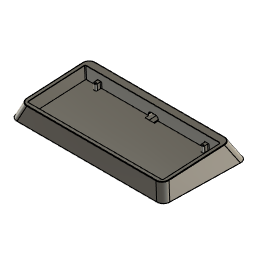
Bruce the Menhir Bottom Mount (Autodesk Fusion 360 design; units mm, degrees)
Autodesk Fusion 360 part; units mm, degrees
sketch "Top Plane Sketch" plane through (0, 0, 0) normal (0, 0, 1) x (1, 0, 0)
  line L0 (-95.25, -40.4812) -> (95.25, -40.4812) construction
  line L1 (95.25, -40.4812) -> (95.25, 40.4812) construction
  line L2 (95.25, 40.4812) -> (-95.25, 40.4812) construction
  line L3 (-95.25, 40.4812) -> (-95.25, -40.4812) construction
  line L4 (-95.75, -40.9812) -> (95.75, -40.9812)
  line L5 (95.75, -40.9812) -> (95.75, 40.9812)
  line L6 (95.75, 40.9813) -> (-95.75, 40.9813)
  line L7 (-95.75, 40.9813) -> (-95.75, -40.9812)
  line L8 (-100.75, -45.9812) -> (100.75, -45.9812)
  line L9 (100.75, -45.9812) -> (100.75, 50.9812)
  line L10 (100.75, 50.9813) -> (-100.75, 50.9813)
  line L11 (-100.75, 50.9813) -> (-100.75, -45.9812)
  line L12 (-95.25, 40.4812) -> (95.25, -40.4812) construction
  line L13 (95.25, 40.4812) -> (-95.25, -40.4812) construction
  circle A0 centre (0, 0) radius 1.8249 construction
  dimension "d1" = 190.5
  dimension "d2" = 80.9625
  dimension "d3" = 0.5
  dimension "d9" = 10
  dimension "d10" = 5
  dimension "d11" = 5
  dimension "d12" = 5
  constraint horizontal L0
  constraint vertical L1
  constraint horizontal L2
  constraint vertical L3
  constraint midpoint L12 A0.centre
  measures "d1" distance of L0.start L0.end
  measures "d2" distance of L0.start L2.end
  measures "d9" distance of L6 L10
  measures "d10" distance of L7 L11
  measures "d11" distance of L5 L9
  measures "d12" distance of L4 L8
ref_plane "WorkPlane1" through (0, 0, -50) normal (0, 0, 1) x (1, 0, 0)
sketch "Base Plane Sketch" plane through (0, 0, -50) normal (0, 0, 1) x (1, 0, 0)
  line L0 (95.25, -40.4813) -> (-95.25, -40.4813) construction
  line L1 (-95.25, -40.4813) -> (-95.25, 40.4812) construction
  line L2 (-95.25, 40.4812) -> (95.25, 40.4812) construction
  line L3 (95.25, 40.4812) -> (95.25, -40.4813) construction
  line L4 (95.25, -40.4813) -> (-95.25, 40.4813) construction
  line L5 (-95.25, -40.4813) -> (95.25, 40.4812) construction
  circle A0 centre (0, 0) radius 6.9017 construction
  line L6 (95.75, -40.9813) -> (-95.75, -40.9813) construction
  line L7 (-95.75, -40.9813) -> (-95.75, 40.9812) construction
  line L8 (-95.75, 40.9812) -> (95.75, 40.9812) construction
  line L9 (95.75, 40.9812) -> (95.75, -40.9812) construction
  line L10 (-100.75, 50.9812) -> (100.75, 50.9812) construction
  line L11 (100.75, 50.9812) -> (100.75, -45.9812) construction
  line L12 (100.75, -45.9813) -> (-100.75, -45.9813) construction
  line L13 (-100.75, -45.9813) -> (-100.75, 50.9812) construction
  line L14 (-120.75, 74.9813) -> (120.75, 74.9813)
  line L15 (120.75, 74.9813) -> (120.75, -65.9813)
  line L16 (120.75, -65.9813) -> (-120.75, -65.9812)
  line L17 (-120.75, -65.9812) -> (-120.75, 74.9812)
  dimension "d14" = 190.5
  dimension "d15" = 80.9625
  dimension "d16" = -0.5
  dimension "d17" = 10
  dimension "d18" = 5
  dimension "d19" = 5
  dimension "d20" = 5
  dimension "d21" = 20
  dimension "d22" = 20
  dimension "d23" = 20
  dimension "d24" = 24
  constraint horizontal L0
  constraint perpendicular L0 L1
  constraint parallel L0 L2
  constraint parallel L1 L3
  constraint coincident L4 A0.centre
  constraint coincident L5 A0.centre
  constraint coincident A0.centre origin
  constraint horizontal L10
  constraint vertical L11
  constraint horizontal L12
  constraint vertical L13
  constraint horizontal L14
  constraint vertical L15
  constraint horizontal L16
  constraint vertical L17
  measures "d14" distance of L1.end L2.end
  measures "d15" distance of L0.end L1.end
  measures "d17" distance of L8 L10
  measures "d18" distance of L7 L13
  measures "d19" distance of L9 L11
  measures "d20" distance of L6 L12
  measures "d21" distance of L12 L16
  measures "d22" distance of L11 L15
  measures "d23" distance of L13 L17
  measures "d24" distance of L10 L14
loft "Loft1" add profiles "Top Plane Sketch", "Base Plane Sketch" section 1 section 2
sketch "Angle Cut Line" plane through (0, -39.639, 15.8556) normal (0, -0.928477, 0.371391) x (1, 0, 0)
  line L0 (100.75, -17.077) -> (-100.75, -17.077)
  line L1 (-100.75, -17.077) -> (-120.75, -70.9287)
  line L2 (-120.75, -70.9287) -> (120.75, -70.9287)
  line L3 (120.75, -70.9287) -> (100.75, -17.077)
  line L4 (-108.5492, -38.077) -> (108.5492, -38.077)
  dimension "d37" = 21
  constraint coincident L1 L4.start
  constraint coincident L3 L4.end
  constraint parallel L2 L4
  measures "d37" distance of L0 L4
ref_plane "WorkPlane2" through (0, -53.7805, -19.498) normal (0, 0.052336, 0.99863) x (1, 0, 0)
extrude "Extrude1" cut 1 faces at (-40.25, 27.9937, -50) along direction (0, 0, -1) up to surface end surface through (0, -53.7805, -19.498) normal (0, 0.052336, 0.99863) offset 0
fillet "Fillet1" radius 10 4 edges at (-105.8766, 57.1332, -12.8166) (-104.6496, -49.8809, -9.749) (104.6496, -49.8809, -9.749) (105.8766, 57.1332, -12.8166)
extrude "Extrude2" cut sketch "Top Plane Sketch" against normal blind 18.06 contours L4 L5 L6 L7
fillet "Fillet2" radius 1 4 edges at (-95.75, 40.9813, -9.03) (95.75, 40.9813, -9.03) (95.75, -40.9812, -9.03) (-95.75, -40.9812, -9.03)
chamfer "Chamfer1" distance 0.5 angle 45 8 edges at (0, -45.9812, 0) (98.1037, -43.335, 0) (100.75, 2.4876, 0) (98.1846, 48.3392, 0) (0, 50.9813, 0) (-98.1846, 48.3392, 0) (-100.75, 2.4876, 0) (-98.1037, -43.335, 0)
chamfer "Chamfer3" distance 0.25 angle 45 8 edges at (0, 40.9813, 0) (95.4571, 40.6884, 0) (95.75, 0, 0) (95.4571, -40.6884, 0) (0, -40.9812, 0) (-95.4571, -40.6884, 0) (-95.75, 0, 0) (-95.4571, 40.6884, 0)
chamfer "Chamfer4" distance 0.5 angle 45 8 edges at (-109.7715, 4.5245, -22.5536) (-105.9572, -51.1885, -19.6338) (0, -53.7805, -19.498) (105.9572, -51.1885, -19.6338) (109.7715, 4.5245, -22.5536) (108.3811, 60.5749, -25.4911) (0, 63.2852, -25.6332) (-108.3811, 60.5749, -25.4911)
sketch "Screw Post Sketch" plane through (0, 0, -18.06) normal (0, 0, 1) x (1, 0, 0)
  arc A0 (-95.75, -39.9812) -> (-94.75, -40.9812) centre (-94.75, -39.9812) ccw
  line L0 (79.45, -40.9812) -> (94.75, -40.9812)
  arc A1 (94.75, -40.9813) -> (95.75, -39.9813) centre (94.75, -39.9813) ccw
  line L1 (95.75, -39.9813) -> (95.75, 39.9813)
  arc A2 (95.75, 39.9812) -> (94.75, 40.9813) centre (94.75, 39.9813) ccw
  line L2 (-79.45, 40.9813) -> (-94.75, 40.9813)
  arc A3 (-94.75, 40.9813) -> (-95.75, 39.9813) centre (-94.75, 39.9813) ccw
  line L3 (-95.75, 39.9813) -> (-95.75, -39.9812)
  arc A4 (-95.75, -39.9812) -> (-94.75, -40.9812) centre (-94.75, -39.9812) ccw
  line L4 (-72.95, -40.9812) -> (72.95, -40.9812)
  arc A5 (94.75, -40.9813) -> (95.75, -39.9813) centre (94.75, -39.9813) ccw
  line L5 (95.75, -39.9813) -> (95.75, 39.9813)
  arc A6 (95.75, 39.9812) -> (94.75, 40.9813) centre (94.75, 39.9813) ccw
  line L6 (72.95, 40.9813) -> (-72.95, 40.9812)
  arc A7 (-94.75, 40.9813) -> (-95.75, 39.9813) centre (-94.75, 39.9813) ccw
  line L7 (-95.75, 39.9813) -> (-95.75, -39.9812)
  arc A8 (-95.75, -39.9812) -> (-94.75, -40.9812) centre (-94.75, -39.9812) ccw
  line L8 (-94.75, -40.9812) -> (94.75, -40.9812)
  arc A9 (94.75, -40.9813) -> (95.75, -39.9813) centre (94.75, -39.9813) ccw
  line L9 (95.75, -39.9813) -> (95.75, 39.9813)
  arc A10 (95.75, 39.9812) -> (94.75, 40.9813) centre (94.75, 39.9813) ccw
  line L10 (94.75, 40.9813) -> (-94.75, 40.9813)
  arc A11 (-94.75, 40.9813) -> (-95.75, 39.9813) centre (-94.75, 39.9813) ccw
  line L11 (-95.75, 39.9813) -> (-95.75, -39.9812)
  line L12 (-95.25, 39.9813) -> (-95.25, -39.9812) construction
  arc A12 (-95.25, -39.9812) -> (-94.75, -40.4812) centre (-94.75, -39.9812) ccw construction
  line L13 (-94.75, -40.4812) -> (94.75, -40.4812) construction
  arc A13 (94.75, -40.4813) -> (95.25, -39.9813) centre (94.75, -39.9813) ccw construction
  line L14 (95.25, -39.9813) -> (95.25, 39.9813) construction
  arc A14 (95.25, 39.9812) -> (94.75, 40.4812) centre (94.75, 39.9813) ccw construction
  line L15 (94.75, 40.4812) -> (-94.75, 40.4813) construction
  arc A15 (-94.75, 40.4813) -> (-95.25, 39.9813) centre (-94.75, 39.9813) ccw construction
  circle A16 centre (-76.2, 35.7187) radius 1
  circle A17 centre (76.2, 35.7187) radius 1
  circle A18 centre (-76.2, -35.7187) radius 1
  circle A19 centre (76.2, -35.7187) radius 1
  circle A20 centre (-76.2, 35.7187) radius 2.25
  circle A21 centre (76.2, 35.7187) radius 2.25
  circle A22 centre (76.2, -35.7187) radius 2.25
  circle A23 centre (-76.2, -35.7187) radius 2.25
  line L16 (-78.45, 35.7187) -> (-78.45, 39.9813)
  line L17 (-73.95, 35.7187) -> (-73.95, 39.9813)
  line L18 (-78.45, -35.7187) -> (-78.45, -39.9812)
  line L19 (-73.95, -35.7187) -> (-73.95, -39.9812)
  line L20 (78.45, -35.7187) -> (78.45, -39.9812)
  line L21 (73.95, -35.7187) -> (73.95, -39.9812)
  line L22 (73.95, 35.7187) -> (73.95, 39.9813)
  line L23 (78.45, 35.7187) -> (78.45, 39.9813)
  arc A24 (-78.45, 39.9813) -> (-79.45, 40.9812) centre (-79.45, 39.9813) ccw
  arc A25 (-72.95, 40.9812) -> (-73.95, 39.9813) centre (-72.95, 39.9813) ccw
  arc A26 (73.95, 39.9813) -> (72.95, 40.9812) centre (72.95, 39.9813) ccw
  arc A27 (79.45, 40.9812) -> (78.45, 39.9813) centre (79.45, 39.9813) ccw
  arc A28 (78.45, -39.9812) -> (79.45, -40.9813) centre (79.45, -39.9812) ccw
  arc A29 (72.95, -40.9812) -> (73.95, -39.9812) centre (72.95, -39.9812) ccw
  arc A30 (-73.95, -39.9812) -> (-72.95, -40.9812) centre (-72.95, -39.9812) ccw
  arc A31 (-79.45, -40.9812) -> (-78.45, -39.9812) centre (-79.45, -39.9813) ccw
  dimension "d80" = 2
  dimension "d81" = 19.05
  dimension "d82" = 2
  dimension "d83" = 2
  dimension "d84" = 2
  dimension "d85" = 19.05
  dimension "d86" = 19.05
  dimension "d87" = 19.05
  dimension "d88" = 4.7625
  dimension "d89" = 4.7625
  dimension "d90" = 4.7625
  dimension "d91" = 4.7625
  dimension "d92" = 4.5
  dimension "d93" = 4.5
  dimension "d94" = 4.5
  dimension "d95" = 4.5
  dimension "d96" = 1
  dimension "d97" = 1
  dimension "d98" = 1
  dimension "d99" = 1
  dimension "d100" = 1
  constraint concentric A16 A20
  constraint concentric A17 A21
  constraint concentric A19 A22
  constraint concentric A18 A23
  constraint coincident A20 L16.start
  constraint tangent A20 L16
  constraint perpendicular L10 L16
  constraint coincident A20 L17.start
  constraint tangent A20 L17
  constraint perpendicular L6 L17
  constraint coincident A23 L18.start
  constraint tangent A23 L18
  constraint perpendicular L4 L18
  constraint coincident A23 L19.start
  constraint tangent A23 L19
  constraint perpendicular L4 L19
  constraint coincident A22 L20.start
  constraint tangent A22 L20
  constraint perpendicular L4 L20
  constraint coincident A22 L21.start
  constraint tangent A22 L21
  constraint perpendicular L0 L21
  constraint coincident A21 L22.start
  constraint tangent A21 L22
  constraint perpendicular L10 L22
  constraint coincident A21 L23.start
  constraint tangent A21 L23
  constraint perpendicular L2 L23
  constraint concentric A0 A12
  constraint concentric A1 A13
  constraint concentric A2 A14
  constraint concentric A3 A15
  constraint tangent A13 L14
  constraint tangent A12 L13
  constraint tangent L12 A15
  constraint tangent L12 A12
  constraint tangent A14 L15
  constraint tangent L13 A13
  constraint tangent L15 A15
  constraint tangent L14 A14
  constraint tangent L2 A24
  constraint tangent L16 A24
  constraint tangent L17 A25
  constraint tangent L6 A25
  constraint equal A24 A25
  constraint tangent L6 A26
  constraint tangent L22 A26
  constraint tangent L23 A27
  constraint tangent L20 A28
  constraint tangent L0 A28
  constraint tangent L21 A29
  constraint tangent L4 A29
  constraint equal A28 A29
  constraint tangent L19 A30
  constraint tangent L4 A30
  constraint equal A28 A30
  constraint tangent L18 A31
  measures "d80" diameter of A16
  measures "d81" distance of L12 A16.centre
  measures "d82" diameter of A17
  measures "d83" diameter of A18
  measures "d84" diameter of A19
  measures "d85" distance of L12 A18.centre
  measures "d86" distance of L14 A19.centre
  measures "d87" distance of L14 A17.centre
  measures "d88" distance of L15 A16.centre
  measures "d89" distance of L15 A17.centre
  measures "d90" distance of L13 A19.centre
  measures "d91" distance of L13 A18.centre
  measures "d92" diameter of A20
  measures "d93" diameter of A21
  measures "d94" diameter of A22
  measures "d95" diameter of A23
  measures "d96" radius of A24
  measures "d97" radius of A26
  measures "d98" radius of A27
  measures "d99" radius of A28
  measures "d100" radius of A31
extrude "Extrude4" add sketch "Screw Post Sketch" along normal blind 8.41 contours L8 A23 L18 L19 A30 A31 | L10 A20 L16 L17 A24 A25 | L8 A22 L20 L21 A28 A29 | A23 | L10 A21 L22 L23 A26 A27 | A20 | A22 | A21
sketch "USB C Hole" plane through (0, 40.9813, 0) normal (0, -1, 0) x (1, 0, 0)
  line L0 (94.75, -0.25) -> (-94.75, -0.25)
  line L1 (-94.75, -0.25) -> (-94.75, -18.06)
  line L2 (94.75, -18.06) -> (94.75, -0.25)
  line L3 (0, -18.06) -> (0, -16.23) construction
  line L4 (6.975, -12.15) -> (-6.975, -12.15)
  line L5 (-6.975, -12.15) -> (-6.975, -20.31)
  line L6 (-6.975, -20.31) -> (6.975, -20.31)
  line L7 (6.975, -20.31) -> (6.975, -12.15)
  line L8 (6.975, -12.15) -> (-6.975, -20.31) construction
  line L9 (-6.975, -12.15) -> (6.975, -20.31) construction
  line L10 (72.95, -9.65) -> (79.45, -9.65)
  line L11 (79.45, -18.06) -> (94.75, -18.06)
  line L12 (-79.45, -18.06) -> (-79.45, -9.65)
  line L13 (-72.95, -9.65) -> (-72.95, -18.06)
  line L14 (-72.95, -18.06) -> (72.95, -18.06)
  line L15 (72.95, -18.06) -> (72.95, -9.65)
  line L16 (79.45, -9.65) -> (79.45, -18.06)
  line L17 (-79.45, -9.65) -> (-72.95, -9.65)
  line L18 (-94.75, -18.06) -> (-79.45, -18.06)
  line L19 (-94.75, -18.06) -> (0, -18.06)
  line L20 (-6.975, -16.23) -> (6.975, -16.23) construction
  point P0 (0, -16.23)
  dimension "d60" = 1.83
  dimension "d61" = 13.95
  dimension "d62" = 8.16
  constraint horizontal L4
  constraint perpendicular L4 L5
  constraint parallel L4 L6
  constraint parallel L5 L7
  constraint coincident L8 P0
  constraint coincident L9 P0
  constraint coincident P0 L3.end
  constraint coincident L1.end L18.start
  constraint midpoint L14 L3.start
  constraint midpoint L5 L20.start
  constraint midpoint L7 L20.end
  constraint perpendicular L3 L20
  constraint coincident L3.start L19.end
  measures "d60" distance of L3.start P0
  measures "d61" distance of L5.end L6.end
  measures "d62" distance of L4.end L5.end
extrude "Extrude5" cut sketch "USB C Hole" along normal blind -25 and the other way blind -5 contours L5 L6 L7 L14 L19 | L4 L5 L7 L14 L19
fillet "Fillet3" radius 3.8 4 edges at (6.975, 48.3557, -20.31) (6.975, 48.8973, -12.15) (-6.975, 48.3557, -20.31) (-6.975, 48.8973, -12.15)
chamfer "Chamfer5" distance 0.25 angle 45 8 edges at (0, 56.8133, -12.15) (-5.862, 57.3475, -13.263) (-6.975, 58.7717, -16.23) (-5.862, 60.1958, -19.197) (0, 60.7301, -20.31) (5.862, 60.1958, -19.197) (6.975, 58.7717, -16.23) (5.862, 57.3475, -13.263)
move_body "Move2" bodies 1 to x (1, 0, 0) y (0, 0.99863, 0.052336) z (0, -0.052336, 0.99863) at (0, -1.0948, 2.7618)
equation "d1 = 19.05 mm * 10"
equation "d2 = 19.05 mm * 4.25"
equation "d14 = 19.05 mm * 10"
equation "d15 = 19.05 mm * 4.25"
equation "d17 = d9"
equation "d18 = d10"
equation "d19 = d11"
equation "d20 = d12"
equation "d21 = 10 mm * 2"
equation "d22 = d21"
equation "d23 = d21"
equation "d24 = 12 mm * 2"
equation "d25 = -3 deg"
equation "d60 = ( 3.66 / 2 ) * 1 mm"
equation "d79 = -d25"
named bodies: "Bruce the Menhir"
